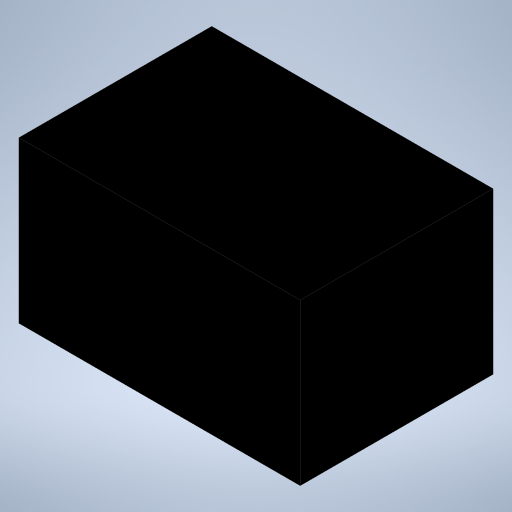
# Autodesk Inventor part: PTC
Saved by Autodesk Inventor 2023 (Build 270158000, 158)
## iProperties
Created: 2023-03-17
Part Number: PTC
Material: Generic
Document SubType Name: Modeling
Designer: kk4764
Density: 1 g/cm^3
Appearance: Default
Author: kk4764
Autodesk Inventor part; units mm, degrees
ref_plane "YZ Plane" through (0, 0, 0) normal (1, 0, 0) x (0, 1, 0)
ref_plane "XZ Plane" through (0, 0, 0) normal (0, 1, 0) x (-1, 0, 0)
ref_plane "XY Plane" through (0, 0, 0) normal (0, 0, 1) x (1, 0, 0)
sketch "Sketch1" plane through (0, 0, 0) normal (0, 0, 1) x (1, 0, 0)
  line L0 (0, 0) -> (889, 0)
  line L1 (889, 0) -> (889, -508)
  line L2 (889, -508) -> (0, -508)
  line L3 (0, -508) -> (0, 0)
  dimension "d0" = 508
  dimension "d1" = 889
  constraints: 8 end point, 2 parallel, 1 horizontal, 1 perpendicular
  measures "d0" distance of L0.end L1.end
  measures "d1" distance of L1.end L2.end
extrude "Extrusion1" add sketch "Sketch1" along normal blind 609.6
body "Solid1"
